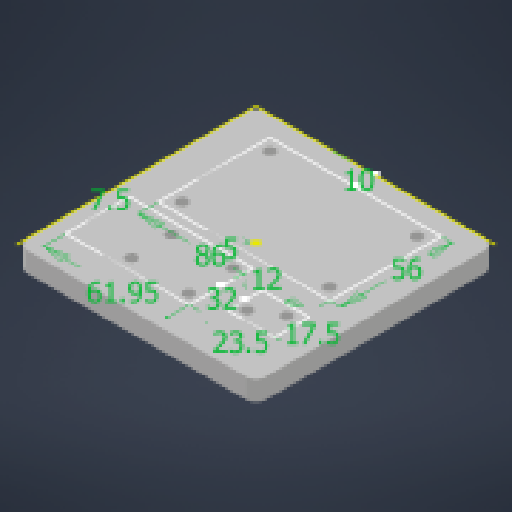
# Autodesk Inventor part: PCB_Housing_01_003
Saved by Autodesk Inventor 2026.2 (Build 302298000, 298)
## iProperties
Created: 2026-02-18
Part Number: PCB_Housing_01_003
Material: Generic
Document SubType Name: Modeling
Designer: vckot
Density: 1 g/cm^3
Appearance: Default
Author: vckot
Autodesk Inventor part; units mm, degrees
ref_plane "YZ Plane" through (0, 0, 0) normal (1, 0, 0) x (0, 1, 0)
ref_plane "XZ Plane" through (0, 0, 0) normal (0, 1, 0) x (-1, 0, 0)
ref_plane "XY Plane" through (0, 0, 0) normal (0, 0, 1) x (1, 0, 0)
sketch "Sketch1" plane through (0, 0, 0) normal (0, 1, 0) x (-1, 0, 0)
  line L0 (-60, 60) -> (60, 60)
  line L1 (60, 60) -> (60, -60)
  line L2 (60, -60) -> (-60, -60)
  line L3 (-60, -60) -> (-60, 60)
  line L4 (-60, 60) -> (60, -60) construction
  line L5 (60, 60) -> (-60, -60) construction
  point P0 (0, 0)
  dimension "d2" = 120
  dimension "d3" = 120
  constraints: 12 end point, 2 midpoint, 2 parallel, 1 horizontal, 1 perpendicular
  measures "d2" distance of L1.end L2.end
  measures "d3" distance of L0.end L1.end
extrude "Extrusion1" add sketch "Sketch1" along normal blind 10
sketch "Sketch2" plane through (0, 10, 0) normal (0, 1, 0) x (1, 0, 0)
  line L0 (-50, -43) -> (6, -43)
  line L1 (6, -43) -> (6, 43)
  line L2 (6, 43) -> (-50, 43)
  line L3 (-50, 43) -> (-50, -43)
  line L4 (-60, 60) -> (-60, -60) projected
  line L5 (-60, -60) -> (60, -60) projected
  line L6 (11, -52.5) -> (43, -52.5)
  line L7 (43, -52.5) -> (43, 9.45)
  line L8 (43, 9.45) -> (11, 9.45)
  line L9 (11, 9.45) -> (11, -52.5)
  line L10 (18.25, 21.45) -> (35.75, 21.45)
  line L11 (35.75, 21.45) -> (35.75, 44.95)
  line L12 (35.75, 44.95) -> (18.25, 44.95)
  line L13 (18.25, 44.95) -> (18.25, 21.45)
  point P0 (0, 0)
  point P1 (27, 21.45)
  point P2 (27, 9.45)
  point P3 (-50, 0)
  point P4 (-60, 0)
  dimension "d4" = 86
  dimension "d5" = 56
  dimension "d6" = 10
  dimension "d8" = 61.95
  dimension "d9" = 32
  dimension "d10" = 5
  dimension "d11" = 7.5
  dimension "d12" = 23.5
  dimension "d13" = 17.5
  dimension "d14" = 12
  constraints: 24 end point, 6 parallel, 4 midpoint, 3 horizontal, 3 perpendicular, 1 horizontal alignment, 1 vertical alignment
  measures "d4" distance of L0.end L1.end
  measures "d5" distance of L1.end L2.end
  measures "d6" distance between parallel lines of L3 L4
  measures "d8" distance of L6.end L7.end
  measures "d9" distance of L7.end L8.end
  measures "d10" distance between parallel lines of L1 L9
  measures "d11" distance between parallel lines of L5 L6
  measures "d12" distance of L10.end L11.end
  measures "d13" distance of L11.end L12.end
  measures "d14" distance between parallel lines of L10 L8
fillet "Fillet1" radius 5 4 edges at (60, 5, -60) (60, 5, 60) (-60, 5, -60) (-60, 5, 60)
sketch "Sketch3" plane through (0, 0, 0) normal (0, -1, 0) x (1, 0, 0)
  circle A0 centre (17, 25.35) radius 3.25 projected
  circle A1 centre (37, 25.35) radius 3.25 projected
  circle A2 centre (0, 37) radius 3.25 projected
  circle A3 centre (-44, 37) radius 3.25 projected
  circle A4 centre (-44, -37) radius 3.25 projected
  circle A5 centre (0, -37) radius 3.25 projected
  circle A6 centre (23.25, -38.7) radius 3.25 projected
  circle A7 centre (30.75, -26.45) radius 3.25 projected
  circle A8 centre (38, -4.45) radius 3.25 projected
  circle A9 centre (16, -4.45) radius 3.25 projected
  point P0 (0, 0)
hole "Hole1" at (37, 0, 25.35) at (38, 0, -4.45) at (30.75, 0, -26.45) at (23.25, 0, -38.7) at (16, 0, -4.45) at (17, 0, 25.35) at (0, 0, 37) at (0, 0, -37) at (-44, 0, -37) at (-44, 0, 37) direction (0, 1, 0) diameter 5.5 end through all counterbore diameter 12.24 counterbore depth 3.65 clearance for "Hex Head Cap Screw" size "M5" standard "Ansi Metric M Profile"
body "Solid1"
